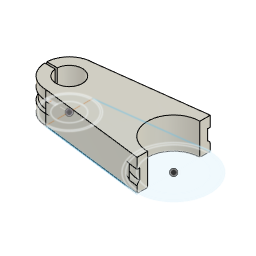
Pole mount (50mm) (Autodesk Fusion 360 design; units mm, degrees)
Autodesk Fusion 360 part; units mm, degrees
sketch "Sketch1" plane through (0, 0, 0) normal (0, 0, 1) x (1, 0, 0)
  circle A0 centre (0, 0) radius 12.5
  circle A1 centre (0, 0) radius 22.5
  circle A2 centre (100, 0) radius 25
  circle A3 centre (100, 0) radius 35
  line L0 (-0.0472, 22.5) -> (-0.0472, -22.5) construction
  line L1 (100, 35) -> (100, -35)
  line L2 (100, -35) -> (-0.0472, -22.5)
  line L3 (100, 35) -> (-0.0472, 22.5)
  line L4 (0, 0) -> (-22.5, 0) construction
  line L5 (-22.4778, 1) -> (-12.4599, 1)
  line L6 (-12.4599, -1) -> (-22.4778, -1)
  line L7 (-18.0009, 0) -> (-18.0009, 1) construction
  line L8 (-18.0009, 0) -> (-18.0009, -1) construction
  circle A4 centre (100, 0) radius 32.5
  circle A5 centre (0, 0) radius 21
  dimension "d1" = 25
  dimension "d2" = 45
  dimension "d3" = 50
  dimension "d4" = 70
  dimension "d5" = 100
  dimension "d6" = 2
  dimension "d9" = 65
  dimension "d21" = 42
  constraint coincident A0.centre A1.centre
  constraint concentric A0 A1
  constraint concentric A2 A3
  constraint coincident A1 L0.start
  constraint coincident A1 L0.end
  constraint vertical L0
  constraint coincident A3 L1.start
  constraint coincident A3 L1.end
  constraint vertical L1
  constraint midpoint A2.centre L1
  constraint coincident A1 L4.end
  constraint perpendicular L0 L4
  constraint coincident A1 L5.start
  constraint coincident A0 L5.end
  constraint perpendicular L0 L5
  constraint coincident A0 L6.start
  constraint coincident A1 L6.end
  constraint parallel L4 L6
  constraint coincident L4 L7.start
  constraint coincident L5 L7.end
  constraint perpendicular L5 L7
  constraint coincident L6 L8.end
  constraint perpendicular L6 L8
  constraint equal L7 L8
  constraint concentric A3 A4
  constraint concentric A0 A5
  measures "d1" diameter of A0
  measures "d2" diameter of A1
  measures "d3" diameter of A2
  measures "d4" diameter of A3
  measures "d5" distance of A0.centre A2.centre
  measures "d6" distance of L5 L6
  measures "d9" diameter of A4
  measures "d21" diameter of A5
extrude "Extrude1" add sketch "Sketch1" along normal blind 30 contours A0 L5 L6 A5 | A1 L5 L6 A5 | A1 A3 L2 L3 | A3 L1 L2 L3 A4 | A2 L1 A4 picked at (-18.0127, -2.0228) picked at (-8.713, 19.6138) picked at (98.3854, -29.879)
extrude "Extrude3" cut sketch "Sketch1" along normal blind 10 from surface at 10 contours A3 L1 L2 L3 A4
fillet "Fillet1" radius 3.75 1 edges at (95.6943, -34.462, 10)
fillet "Fillet2" radius 3.75 1 edges at (95.6943, 34.462, 10)
extrude "Extrude4" cut sketch "Sketch1" along normal mid plane 10 from surface at 15 contours A1 L5 L6 A5 picked at (-8.713, 19.6138)
fillet "Fillet3" radius 1 2 edges at (-15.5694, 16.2433, 20) (-15.5694, -16.2433, 20)
fillet "Fillet4" radius 2.5 1 edges at (21, 0, 10)
